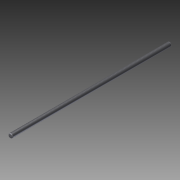
# Autodesk Inventor part: S2_ZSCREW
Saved by Autodesk Inventor 2014 (Build 180170000, 170)
## iProperties
Created: 2011-09-26
Part Number: S2_ZSCREW
Document SubType Name: Modeling
Designer: ERF
Density: 1 g/cm^3
Description: Metric Class 8.8 Plain Steel Threaded Rod M8 Size, 1 Meter Length, 1.25 mm Pitch
Material: Generic
Stock Number: 99055A125
Vendor: McMasterCarr
Project: Shapeoko
Mass: 10.0531 g
Surface Area: 51.2708 cm^2
Volume: 10.0531 cm^3
Appearance: Steel
Title: Threaded Rod
Author: ERF
Autodesk Inventor part; units mm, degrees
ref_plane "YZ Plane" through (0, 0, 0) normal (1, 0, 0) x (0, 1, 0)
ref_plane "XZ Plane" through (0, 0, 0) normal (0, 1, 0) x (-1, 0, 0)
ref_plane "XY Plane" through (0, 0, 0) normal (0, 0, 1) x (1, 0, 0)
sketch "Sketch1" plane through (0, 0, 0) normal (0, 0, 1) x (1, 0, 0)
  circle A0 centre (0, 0) radius 4
  dimension "d0" = 8
  constraints: 1 centre point
  measures "d0" diameter of A0
extrude "Extrusion1" add sketch "Sketch1" along normal blind 300
thread "Thread1" size "M8x1.25" class "6g" standard "ANSI Metric M Profile" full length
fillet "Fillet1" radius 1.5875 2 edges at (-4, 0, 0) (-4, 0, 300)
body "Solid1"
